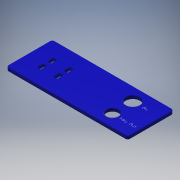
# Autodesk Inventor part: KeyerFront_Iambic
Saved by Autodesk Inventor 2016 (Build 200138000, 138)
## iProperties
Created: 2016-06-11
Part Number: KeyerFront_Iambic
Material: Generic
Document SubType Name: Modeling
Designer: Tyler
Density: 1 g/cm^3
Appearance: Smooth - Navy
Categories: <MemberInstance><Categories><Category DisplayName="" Mnemonic="CABLEANDHARNESS" InternalName="e4a7e005-5e42-4d16-b293-125e7f0d0512"><Category DisplayName="" Mnemonic="CONNECTORS" InternalName="6f634eba-a678-4820-a31d-2c2d5ee6728e"><CategoryParameter DisplayName="" Mnemonic="REFDES" InternalName="c3740e8c-60ab-4d5d-8584-52b73222f2f0"/><Category DisplayName="" Mnemonic="DISCRETEWIRE" InternalName="9a3407de-09b2-4cdb-8c40-9708d5144a28"/></Category></Category></Categories><FamilyTemplate><FamilyTemplateParameters></FamilyTemplateParameters></FamilyTemplate><CategoryParameterMap><ParamToTemplateMap><ParamToTemplate CategoryParameter="//CategoryParameter[@InternalName='c3740e8c-60ab-4d5d-8584-52b73222f2f0']" ConstantValue=""/></ParamToTemplateMap></CategoryParameterMap></MemberInstance>
Author: Tyler
Autodesk Inventor part; units mm, degrees
ref_plane "YZ Plane" through (0, 0, 0) normal (1, 0, 0) x (0, 1, 0)
ref_plane "XZ Plane" through (0, 0, 0) normal (0, 1, 0) x (-1, 0, 0)
ref_plane "XY Plane" through (0, 0, 0) normal (0, 0, 1) x (1, 0, 0)
sketch "Sketch1" plane through (0, 0, 0) normal (0, 0, 1) x (1, 0, 0)
  line L0 (-29.75, -11.25) -> (29.75, -11.25)
  line L1 (29.75, -11.25) -> (29.75, 11.25)
  line L2 (29.75, 11.25) -> (-29.75, 11.25)
  line L3 (-29.75, 11.25) -> (-29.75, -11.25)
  line L4 (-29.75, -11.25) -> (29.75, 11.25) construction
  line L5 (29.75, -11.25) -> (-29.75, 11.25) construction
  point P0 (0, 0)
  dimension "d0" = 59.5
  dimension "d1" = 22.5
  constraints: 12 end point, 2 midpoint, 2 parallel, 1 horizontal, 1 perpendicular
  measures "d0" distance of L2.end L1.end
  measures "d1" distance of L1.end L0.end
extrude "Extrusion1" add sketch "Sketch1" against normal blind 1.6
fillet "Fillet1" radius 1 4 edges at (29.75, 11.25, -0.8) (-29.75, 11.25, -0.8) (29.75, -11.25, -0.8) (-29.75, -11.25, -0.8)
sketch "Sketch2" plane through (0, 0, 0) normal (0, 0, 1) x (1, 0, 0)
  line L0 (-21.9, 4.1) -> (-20.1, 4.1)
  line L1 (-20.1, 4.1) -> (-20.1, 0.9)
  line L2 (-20.1, 0.9) -> (-21.9, 0.9)
  line L3 (-21.9, 0.9) -> (-21.9, 4.1)
  line L4 (-21.9, 4.1) -> (-20.1, 0.9) construction
  line L5 (-20.1, 4.1) -> (-21.9, 0.9) construction
  line L6 (-20.1, -0.9) -> (-21.9, -0.9)
  line L7 (-21.9, -0.9) -> (-21.9, -4.1)
  line L8 (-21.9, -4.1) -> (-20.1, -4.1)
  line L9 (-20.1, -4.1) -> (-20.1, -0.9)
  line L10 (-20.1, -0.9) -> (-21.9, -4.1) construction
  line L11 (-21.9, -0.9) -> (-20.1, -4.1) construction
  line L12 (-17, 0) -> (-17, 5.3945) construction
  line L13 (-12.1, 4.1) -> (-13.9, 4.1)
  line L14 (-13.9, 4.1) -> (-13.9, 0.9)
  line L15 (-13.9, 0.9) -> (-12.1, 0.9)
  line L16 (-12.1, 0.9) -> (-12.1, 4.1)
  line L17 (-12.1, 4.1) -> (-13.9, 0.9) construction
  line L18 (-13.9, 4.1) -> (-12.1, 0.9) construction
  line L19 (-13.9, -0.9) -> (-12.1, -0.9)
  line L20 (-12.1, -0.9) -> (-12.1, -4.1)
  line L21 (-12.1, -4.1) -> (-13.9, -4.1)
  line L22 (-13.9, -4.1) -> (-13.9, -0.9)
  line L23 (-13.9, -0.9) -> (-12.1, -4.1) construction
  line L24 (-12.1, -0.9) -> (-13.9, -4.1) construction
  line L25 (-29.75, 10.25) -> (-29.75, -10.25) projected
  line L26 (-28.75, -11.25) -> (28.75, -11.25) projected
  point P0 (0, 0)
  point P1 (-21, 2.5)
  point P2 (-21, -2.5)
  point P3 (-13, 2.5)
  point P4 (-13, -2.5)
  dimension "d5" = 17
  dimension "d6" = 1.8
  dimension "d7" = 0.9
  dimension "d8" = 0
  dimension "d10" = 1.8
  dimension "d11" = 1.8
  dimension "d12" = 3.2
  dimension "d13" = 3.2
  dimension "d16" = 4
  dimension "d17" = 8.75
  dimension "d28" = 11.25
  dimension "d29" = 16.75
  constraints: 50 end point, 10 symmetric about line, 8 midpoint, 5 parallel, 2 horizontal, 2 perpendicular, 1 collinear
  measures "d5" distance of L12.start point (0, 0)
  measures "d6" distance between parallel lines of L6 L2
  measures "d7" distance from line of L12.start L2
  measures "d8" vertical distance of point (0, 0) L12.start
  measures "d10" distance of L0.start L0.end
  measures "d11" distance of L6.start L6.end
  measures "d12" distance of L0.end L1.end
  measures "d13" distance of L8.end L6.start
  measures "d16" distance from line of point (-21, 2.5) L12
  measures "d17" distance from line of point (-21, 2.5) L25
  measures "d28" distance from line of L12.start L26
  measures "d29" distance from line of L25 point (-13, 2.5)
extrude "Extrusion2" cut sketch "Sketch2" against normal blind 1.6
sketch "Sketch3" plane through (0, 0, 0) normal (0, 0, 1) x (1, 0, 0)
  line L0 (-29.75, 10.25) -> (-29.75, -10.25) construction
  line L1 (16, 5) -> (16, -5) construction
  circle A0 centre (16, 5) radius 3.5
  circle A1 centre (16, -5) radius 3
  line L2 (-28.75, -11.25) -> (28.75, -11.25) projected
  point P0 (0, 0)
  dimension "d18" = 7
  dimension "d19" = 6
  dimension "d20" = 10
  dimension "d21" = 5
  dimension "d22" = 16
  dimension "d25" = 45.75
  dimension "d26" = 6.25
  dimension "d27" = 16.25
  constraints: 2 centre point, 2 coincident, 2 end point, 1 parallel
  measures "d18" diameter of A0
  measures "d19" diameter of A1
  measures "d20" distance of L1.start L1.end
  measures "d21" vertical distance of point (0, 0) L1.start
  measures "d22" distance from line of L1 point (0, 0)
  measures "d25" distance between parallel lines of L1 L0
  measures "d26" distance from line of L2 L1.end
  measures "d27" distance from line of L2 L1.start
extrude "Extrusion3" cut sketch "Sketch3" against normal through all
sketch "Sketch4" plane through (0, 0, 0) normal (0, 0, 1) x (1, 0, 0)
  line L0 (-29.75, 11.25) -> (29.75, 11.25) construction
  line L1 (29.75, 11.25) -> (29.75, -11.2319) construction
  line L2 (29.75, -11.2319) -> (-29.75, -11.2319) construction
  line L3 (-29.75, -11.2319) -> (-29.75, 11.25) construction
  line L4 (28.75, 11.25) -> (-28.75, 11.25) projected
  line L5 (-29.75, 10.25) -> (-29.75, -10.25) projected
  line L6 (29.75, -10.25) -> (29.75, 10.25) projected
  point P0 (0, 0)
  constraints: 3 collinear, 2 other
decal "Decal1"
sketch "Sketch5" plane through (0, 0, -1.6) normal (0, 0, -1) x (-1, 0, 0)
  line L0 (-29.75, 11.25) -> (29.75, 11.25) construction
  line L1 (29.75, 11.25) -> (29.75, -11.2319) construction
  line L2 (29.75, -11.2319) -> (-29.75, -11.2319) construction
  line L3 (-29.75, -11.2319) -> (-29.75, 11.25) construction
  line L4 (28.75, 11.25) -> (-28.75, 11.25) projected
  line L5 (-29.75, 10.25) -> (-29.75, -10.25) projected
  line L6 (29.75, -10.25) -> (29.75, 10.25) projected
  point P0 (0, 0)
  constraints: 3 collinear, 2 other
decal "Decal2"
equation "\"d7\" = 0.5 * d6"
equation "\"d21\" = 0.5 * d20"
body "Solid1"
